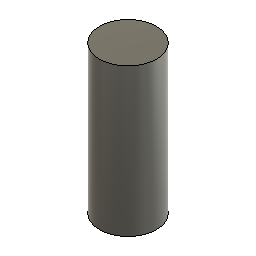
Head Pin (Autodesk Fusion 360 design; units mm, degrees)
Autodesk Fusion 360 part; units mm, degrees
sketch "head Pin Sketch" plane through (0, 0, 0) normal (0, 1, 0) x (1, 0, 0)
  circle A0 centre (0, 0) radius 3.85
  dimension "d602" = 7.7
  constraint coincident A0.centre origin
  measures "d602" diameter of A0
extrude "Extrude1" add sketch "head Pin Sketch" along normal mid plane 20
named bodies: "head Pin"
